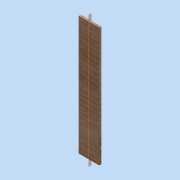
# Autodesk Inventor part: etage-bras
Saved by Autodesk Inventor 2017 (Build 210142000, 142)
## iProperties
Created: 2018-04-01
Part Number: etage-bras
Material: Generic
Document SubType Name: Modeling
Designer: franc
Density: 1 g/cm^3
Appearance: Default
Author: franc
Autodesk Inventor part; units mm, degrees
ref_plane "YZ Plane" through (0, 0, 0) normal (1, 0, 0) x (0, 1, 0)
ref_plane "XZ Plane" through (0, 0, 0) normal (0, 1, 0) x (-1, 0, 0)
ref_plane "XY Plane" through (0, 0, 0) normal (0, 0, 1) x (1, 0, 0)
sketch "Esquisse1" plane through (0, 0, 0) normal (0, 1, 0) x (-1, 0, 0)
  line L0 (57.703, 92.8408) -> (7.703, 92.8408)
  line L1 (7.703, 92.8408) -> (7.703, -197.1592)
  line L2 (7.703, -197.1592) -> (57.703, -197.1592)
  line L3 (57.703, -197.1592) -> (57.703, 92.8408)
  point P0 (0, 0)
  dimension "d0" = 290
  dimension "d1" = 50
  constraints: 8 end point, 2 parallel, 1 horizontal, 1 perpendicular
  measures "d0" distance of L2.end L0.start
  measures "d1" distance of L0.start L0.end
extrude "Extrusion1" add sketch "Esquisse1" along normal blind 5
ref_plane "Plan de construction1" through (-32.703, 0, -197.1592) normal (-1, 0, 0) x (0, 0, 1)
